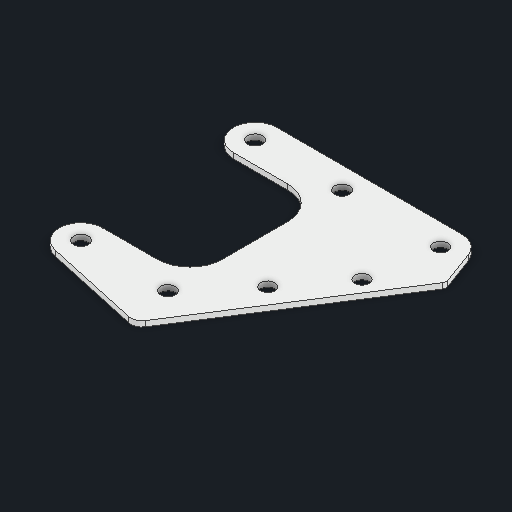
# Autodesk Inventor part: Funnel Gusset V2
Saved by Autodesk Inventor 2025.1 (Build 291241000, 241)
## iProperties
Created: 2024-10-12
Part Number: Funnel Gusset V2
Material: Acetal Resin, White
Document SubType Name: Modeling
Designer: Averey Ku
Density: 1.425 g/cm^3
Appearance: Smooth - White
Mass: 4.93304 g
Surface Area: 49.3118 cm^2
Volume: 3.46178 cm^3
d0: 0.164 in
d1: 0.500 in
d6: 0.375 in
d9: 0.063 in
d17: 0.125 in
Author: Averey Ku
Autodesk Inventor part; units mm, degrees
ref_plane "YZ Plane" through (0, 0, 0) normal (1, 0, 0) x (0, 1, 0)
ref_plane "XZ Plane" through (0, 0, 0) normal (0, 1, 0) x (-1, 0, 0)
ref_plane "XY Plane" through (0, 0, 0) normal (0, 0, 1) x (1, 0, 0)
sketch "main" plane through (0, 0, 0) normal (0, 0, 1) x (1, 0, 0)
  circle A0 centre (-18.8876, -16.6215) radius 2.0828
  arc A1 (-24.8433, -18.8241) -> (-18.8876, -22.9715) centre (-18.8876, -16.6215) ccw
  line L0 (5.6124, 45.0726) -> (-28.2078, -7.9145)
  circle A2 centre (9.8531, -16.6215) radius 2.1844
  line L1 (-18.8876, -22.9715) -> (35.2506, -22.9715)
  line L2 (9.8531, 18.3035) -> (9.8531, -0.7465)
  arc A3 (9.8531, -0.7465) -> (19.3781, -10.2715) centre (19.3781, -0.7465) ccw
  circle A4 centre (9.8531, 34.1785) radius 2.1844
  line L3 (35.2481, -10.2715) -> (19.3781, -10.2715)
  arc A5 (35.2506, -22.9715) -> (35.2481, -10.2715) centre (35.2506, -16.6215) ccw
  circle A6 centre (35.2531, 34.1785) radius 2.1844
  arc A7 (35.2531, 27.8285) -> (36.6181, 40.3801) centre (35.2531, 34.1785) ccw
  circle A8 centre (35.2506, -16.6215) radius 2.1844
  line L4 (-28.3586, -9.3193) -> (-24.8433, -18.8241)
  line L5 (19.3781, 27.8285) -> (35.2531, 27.8285)
  arc A9 (19.3781, 27.8285) -> (9.8531, 18.3035) centre (19.3781, 18.3035) ccw
  arc A10 (-28.2078, -7.9145) -> (-28.3586, -9.3193) centre (-26.8697, -8.7686) ccw
  line L6 (8.9712, 46.4651) -> (36.6181, 40.3801)
  arc A11 (8.9712, 46.4651) -> (5.6124, 45.0726) centre (8.2887, 43.3643) ccw
  circle A12 centre (-3.7188, 18.6506) radius 2.0955
  circle A13 centre (-15.5942, 2.9958) radius 2.0955
  point P0 (9.379, 13.4106)
  point P1 (9.8531, 27.8285)
  dimension "d0" = 4.1656
  dimension "d1" = 12.7
  dimension "d6" = 9.525
  dimension "d9" = 1.5875
  dimension "d17" = 3.175
  dimension "d18" = 50.8
  dimension "d19" = 7.8528
  dimension "d21" = 6.35
  dimension "d22" = 36.7228
  dimension "d23" = 50.8
  dimension "d24" = 25.4
  dimension "d28" = 4.191
  dimension "d29" = 4.191
  measures "d0" diameter of A0
  measures "d1" diameter of A1
  measures "d6" radius of A9
  measures "d9" radius of A10
  measures "d17" radius of A11
  measures "d18" distance of A6.centre A8.centre
  measures "d19" vertical distance of A10.centre A0.centre
  measures "d21" radius of A5
  measures "d22" distance from line of A10.centre L2
  measures "d23" distance of A4.centre A2.centre
  measures "d24" distance from line of A6.centre L2
  measures "d28" diameter of A12
  measures "d29" diameter of A13
sketch "Sketch1" plane through (0, 0, 0) normal (0, 1, 0) x (-1, 0, 0)
  circle A0 centre (-54.1407, -50.8) radius 2.0828
  arc A1 (-60.0964, -53.0027) -> (-54.1407, -57.15) centre (-54.1407, -50.8) ccw
  line L0 (-29.6407, 10.894) -> (-63.461, -42.0931)
  circle A2 centre (-25.4, -50.8) radius 2.1844
  line L1 (-54.1407, -57.15) -> (-0.0025, -57.15)
  line L2 (-25.4, -15.875) -> (-25.4, -34.925)
  arc A3 (-25.4, -34.925) -> (-15.875, -44.45) centre (-15.875, -34.925) ccw
  circle A4 centre (-25.4, 0) radius 2.1844
  line L3 (-0.005, -44.45) -> (-15.875, -44.45)
  arc A5 (-0.0025, -57.15) -> (-0.005, -44.45) centre (-0.0025, -50.8) ccw
  circle A6 centre (0, 0) radius 2.1844
  arc A7 (0, -6.35) -> (1.3649, 6.2016) centre (0, 0) ccw
  circle A8 centre (-0.0025, -50.8) radius 2.1844
  line L4 (-63.6118, -43.4979) -> (-60.0964, -53.0027)
  line L5 (-15.875, -6.35) -> (0, -6.35)
  arc A9 (-15.875, -6.35) -> (-25.4, -15.875) centre (-15.875, -15.875) ccw
  arc A10 (-63.461, -42.0931) -> (-63.6118, -43.4979) centre (-62.1228, -42.9472) ccw
  line L6 (-26.2819, 12.2866) -> (1.3649, 6.2016)
  arc A11 (-26.2819, 12.2866) -> (-29.6407, 10.894) centre (-26.9644, 9.1858) ccw
  circle A12 centre (-38.9719, -15.5279) radius 2.0955
  circle A13 centre (-50.8473, -31.1828) radius 2.0955
  constraints: 1 other
extrude "Extrusion1" add sketch "Sketch1" along normal blind 1.5875
body "Solid1"
